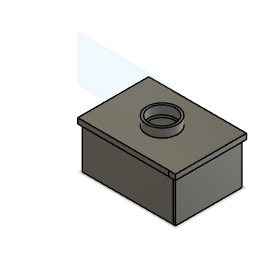
Owl Orb of Protection v5 (Autodesk Fusion 360 design; units mm, degrees)
Autodesk Fusion 360 part; units mm, degrees
sketch "Sketch1" plane through (0, 0, 0) normal (0, 0, 1) x (1, 0, 0)
  line L0 (0, 0) -> (115, 0)
  line L1 (115, 0) -> (115, 55)
  line L2 (115, 55) -> (0, 55)
  line L3 (0, 55) -> (0, 0)
  dimension "d1" = 115
  dimension "d2" = 55
  constraint horizontal L0
  constraint vertical L1
  constraint horizontal L2
  constraint vertical L3
  constraint coincident L0.start L3.end
  measures "d1" distance of L0.start L0.end
  measures "d2" distance of L0.start L2.end
extrude "Extrude1" add sketch "Sketch1" along normal blind 3 makes body 1
sketch "Sketch2" plane through (115, 0, 0) normal (1, 0, 0) x (0, 0, -1)
  line L0 (0, 0) -> (0, 55)
  line L1 (0, 55) -> (-3, 55)
  line L2 (-3, 55) -> (-3, 0)
  line L3 (-3, 0) -> (0, 0)
  line L4 (0, 0) -> (80, 0)
  line L5 (80, 0) -> (80, 55)
  line L6 (80, 55) -> (0, 55)
  line L7 (0, 55) -> (0, 0)
  dimension "d5" = 80
  constraint horizontal L4
  constraint vertical L5
  constraint horizontal L6
  constraint vertical L7
  constraint coincident L0.start L3.end
  measures "d5" distance of L0.start L4.end
extrude "Extrude2" add sketch "Sketch2" along normal blind 3 bodies 1
sketch "Sketch3" plane through (0, 0, -80) normal (0, 0, -1) x (-1, 0, 0)
  line L0 (-115, 0) -> (-115, 55)
  line L1 (-115, 55) -> (-118, 55)
  line L2 (-118, 55) -> (-118, 0)
  line L3 (-118, 0) -> (-115, 0)
  line L4 (-118, 0) -> (0, 0)
  line L5 (0, 0) -> (0, 55)
  line L6 (0, 55) -> (-118, 55)
  line L7 (-118, 55) -> (-118, 0)
  constraint horizontal L4
  constraint vertical L5
  constraint horizontal L6
  constraint vertical L7
  constraint coincident L2.end L3.start
extrude "Extrude3" add sketch "Sketch3" along normal blind 3 separate body contours L0 L4 L5 L6 makes body 2
sketch "Sketch4" plane through (0, 0, 0) normal (-1, 0, 0) x (0, 0, 1)
  line L0 (-80, 0) -> (-80, 55)
  line L1 (-80, 55) -> (-83, 55)
  line L2 (-83, 55) -> (-83, 0)
  line L3 (-83, 0) -> (-80, 0)
  line L4 (-83, 55) -> (3.175, 55)
  line L5 (3.175, 55) -> (3.175, 0)
  line L6 (3.175, 0) -> (-83, 0)
  line L7 (-83, 0) -> (-83, 55)
  constraint horizontal L4
  constraint vertical L5
  constraint horizontal L6
  constraint vertical L7
  constraint coincident L1.end L2.start
extrude "Extrude4" add sketch "Sketch4" along normal blind 3 contours L0 L4 L5 L6 bodies 1 2
extrude "Extrude5" add 2 faces at (-1, 18.3333, -80) (117, 18.3333, -80) along direction (0, 0, -1) blind 3 on bodies 1 bodies 1
sketch "Sketch5" plane through (0, 55, 0) normal (0, 1, 0) x (-1, 0, 0)
  line L0 (-115, -80) -> (-115, 0)
  line L1 (-115, 0) -> (0, 0)
  line L2 (0, 0) -> (0, -80)
  line L3 (0, -80) -> (-115, -80)
  line L4 (-118, 3) -> (-118, -83)
  line L5 (-118, -83) -> (3, -83)
  line L6 (3, -83) -> (3, 3.175)
  line L7 (3, 3.175) -> (0, 3.175)
  line L8 (0, 3.175) -> (0, 3)
  line L9 (0, 3) -> (-118, 3)
  line L10 (3, -83) -> (-118, -83)
  line L11 (-118, -83) -> (-118, 3)
  line L12 (-118, 3) -> (3, 3)
  line L13 (3, 3) -> (3, -83)
  constraint horizontal L10
  constraint vertical L11
  constraint horizontal L12
  constraint vertical L13
  constraint coincident L4.start L9.end
  constraint coincident L5.end L6.start
extrude "Extrude6" add sketch "Sketch5" along normal blind 3 contours L0 L1 L2 L3 | L4 L5 L6 L9 L10 L11 L12 L13 bodies 1
sketch "Sketch6" plane through (0, 58, 0) normal (0, 1, 0) x (-1, 0, 0)
  line L0 (3, 3) -> (-118, 3)
  line L1 (-118, 3) -> (-118, -83)
  line L2 (-118, -83) -> (3, -83)
  line L3 (3, -83) -> (3, 3)
  line L4 (-4.7625, -76.2) -> (-20.6375, -76.2)
  line L5 (-20.6375, -76.2) -> (-20.6375, -3.175)
  line L6 (-20.6375, -3.175) -> (-4.7625, -3.175)
  line L7 (-4.7625, -3.175) -> (-4.7625, -76.2)
  line L8 (-27.3845, -3.175) -> (-27.3845, -76.2)
  line L9 (-43.2595, -3.175) -> (-27.3845, -3.175)
  line L10 (-43.2595, -76.2) -> (-43.2595, -3.175)
  line L11 (-27.3845, -76.2) -> (-43.2595, -76.2)
  line L12 (-50.0065, -3.175) -> (-50.0065, -76.2)
  line L13 (-65.8815, -3.175) -> (-50.0065, -3.175)
  line L14 (-65.8815, -76.2) -> (-65.8815, -3.175)
  line L15 (-50.0065, -76.2) -> (-65.8815, -76.2)
  line L16 (-72.6285, -3.175) -> (-72.6285, -76.2)
  line L17 (-88.5035, -3.175) -> (-72.6285, -3.175)
  line L18 (-88.5035, -76.2) -> (-88.5035, -3.175)
  line L19 (-72.6285, -76.2) -> (-88.5035, -76.2)
  line L20 (-95.2505, -3.175) -> (-95.2505, -76.2)
  line L21 (-111.1255, -3.175) -> (-95.2505, -3.175)
  line L22 (-111.1255, -76.2) -> (-111.1255, -3.175)
  line L23 (-95.2505, -76.2) -> (-111.1255, -76.2)
  dimension "d18" = -90.488
  dimension "d19" = 0
  constraint horizontal L4
  constraint vertical L5
  constraint horizontal L6
  constraint vertical L7
extrude "Extrude7" cut sketch "Sketch6" against normal blind 71.438 contours L4 L5 L6 L7 | L8 L9 L10 L11 | L12 L13 L14 L15 | L16 L17 L18 L19 | L20 L21 L22 L23 bodies 1
sketch "Sketch7" plane through (0, 0, -83) normal (0, 0, -1) x (-1, 0, 0)
  line L0 (-118, 0) -> (3, 0)
  line L1 (3, 0) -> (3, 58)
  line L2 (3, 58) -> (-118, 58)
  line L3 (-118, 58) -> (-118, 0)
sketch "Sketch8" plane through (0, 0, 0) normal (0, -1, 0) x (1, 0, 0)
  line L0 (118, -83) -> (118, 3)
  line L1 (118, 3) -> (0, 3)
  line L2 (0, 3) -> (0, 3.175)
  line L3 (0, 3.175) -> (-3, 3.175)
  line L4 (-3, 3.175) -> (-3, -83)
  line L5 (-3, -83) -> (118, -83)
  line L6 (115, -80) -> (0, -80)
  line L7 (0, -80) -> (0, 0)
  line L8 (0, 0) -> (115, 0)
  line L9 (115, 0) -> (115, -80)
  circle A0 centre (57.5, -40) radius 20
  circle A1 centre (57.5, -40) radius 17
  dimension "d22" = 40
  dimension "d23" = -3
  measures "d22" diameter of A0
extrude "Extrude8" add sketch "Sketch8" along normal blind 14.288 separate body contours A0 makes body 3
sketch "Sketch9" plane through (0, 0, 0) normal (0, -1, 0) x (1, 0, 0)
  line L0 (118, -83) -> (118, 3)
  line L1 (118, 3) -> (0, 3)
  line L2 (0, 3) -> (0, 3.175)
  line L3 (0, 3.175) -> (-3, 3.175)
  line L4 (-3, 3.175) -> (-3, -83)
  line L5 (-3, -83) -> (118, -83)
  line L6 (115, -80) -> (0, -80)
  line L7 (0, -80) -> (0, 0)
  line L8 (0, 0) -> (115, 0)
  line L9 (115, 0) -> (115, -80)
  line L10 (118, 3) -> (0, 3)
  line L11 (0, 3) -> (0, -80)
  line L12 (0, -80) -> (118, -80)
  line L13 (118, -80) -> (118, 3)
  constraint horizontal L10
  constraint vertical L11
  constraint horizontal L12
  constraint vertical L13
  constraint coincident L6.end L7.start
  constraint coincident L0.end L1.start
extrude "Extrude9" add sketch "Sketch9" along normal blind 3 separate body makes body 4
combine "Combine1" operation add target body 4 tool bodies 3
sketch "Sketch10" plane through (0, -3, 0) normal (0, -1, 0) x (1, 0, 0)
  line L0 (118, -83) -> (118, 3)
  line L1 (118, 3) -> (0, 3)
  line L2 (0, 3) -> (0, 3.175)
  line L3 (0, 3.175) -> (-3, 3.175)
  line L4 (-3, 3.175) -> (-3, -83)
  line L5 (-3, -83) -> (118, -83)
  circle A0 centre (57.5, -40) radius 20
  line L6 (121, 6) -> (3, 6)
  line L7 (3, 6) -> (3, 6.175)
  line L8 (3, 6.175) -> (-6, 6.175)
  line L9 (-6, 6.175) -> (-6, -86)
  line L10 (-6, -86) -> (121, -86)
  line L11 (121, -86) -> (121, 6)
  dimension "d28" = 3
extrude "Extrude10" add sketch "Sketch10" against normal blind 5 separate body contours L6 L7 L8 L9 L10 L11 makes body 5
combine "Combine2" operation add target body 4 tool bodies 5
extrude "Extrude11" add 1 faces at (77.6667, 2, -85) along direction (0, 1, 0) blind 2 on bodies 4 bodies 4
sketch "Sketch11" plane through (0, -3, 0) normal (0, -1, 0) x (1, 0, 0)
  circle A0 centre (57.5, -40) radius 17
  circle A1 centre (57.5, -40) radius 17
  constraint concentric A0 A1
extrude "Extrude12" cut sketch "Sketch11" against normal blind 47.625 bodies 4
split "Split1" by plane through (0, -3, 0) normal (0, -1, 0) bodies 4 makes body 6 at (77.4006, -6.7627, -38.0086)
move_body "Move1" bodies 4 6 1 to x (-1, 0, 0) y (0, -1, 0) z (0, 0, 1) at (206.376, 113, 0)
move_body "Move2" bodies 6 4 1 to x (1, 0, 0) y (0, 1, 0) z (0, 0, 1) at (0, -65.0875, 0)
named bodies: "orbcase", "orblid", "Toporblid (1)"
